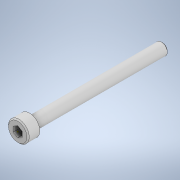
# Autodesk Inventor part: sruba
Saved by Autodesk Inventor 2020 (Build 240168000, 168)
## iProperties
Created: 2020-03-28
Part Number: sruba
Material: Ogólny
Document SubType Name: Modeling
Designer: niedz
Density: 1 g/cm^3
Appearance: Domyślna
Author: niedz
Autodesk Inventor part; units mm, degrees
ref_plane "YZ Plane" through (0, 0, 0) normal (1, 0, 0) x (0, 1, 0)
ref_plane "XZ Plane" through (0, 0, 0) normal (0, 1, 0) x (-1, 0, 0)
ref_plane "XY Plane" through (0, 0, 0) normal (0, 0, 1) x (1, 0, 0)
sketch "Szkic1" plane through (0, 0, 0) normal (0, 0, 1) x (1, 0, 0)
  circle A0 centre (0, 0) radius 3.5
  dimension "d0" = 7
  constraints: 1 centre point, 1 coincident
  measures "d0" diameter of A0
extrude "Wyciągnięcie proste1" add sketch "Szkic1" along normal blind 4
chamfer "Faza1" distance 0.4 angle 45 1 edges at (-3.5, 0, 4)
sketch "Szkic2" plane through (0, 0, 4) normal (0, 0, 1) x (1, 0, 0)
  point P0 (0, 0)
sketch "Szkic3" plane through (0, 0, 4) normal (0, 0, 1) x (1, 0, 0)
  circle A0 centre (0, 0) radius 1.5355
  line L0 (1.5355, 0) -> (1.5355, 0.8865)
  line L1 (1.5355, 0) -> (1.5355, -0.8865)
  line L2 (0.7677, -1.3298) -> (1.5355, -0.8865)
  line L3 (0.7677, -1.3298) -> (0, -1.773)
  line L4 (0.7678, 1.3298) -> (0, 1.773)
  line L5 (-0.7677, 1.3298) -> (0, 1.773)
  line L6 (-1.5355, 0) -> (-1.5355, 0.8865)
  line L7 (-0.7677, 1.3298) -> (-1.5355, 0.8865)
  line L8 (-0.7678, -1.3298) -> (0, -1.773)
  line L9 (0.7678, 1.3298) -> (1.5355, 0.8865)
  line L10 (-1.5355, 0) -> (-1.5355, -0.8865)
  line L11 (-0.7678, -1.3298) -> (-1.5355, -0.8865)
  dimension "d6" = 3.071
  constraints: 24 end point, 4 vertical, 1 coincident, 1 horizontal alignment, 1 point on line, 4 other
extrude "Wyciągnięcie proste2" cut sketch "Szkic3" against normal blind 2
sketch "Szkic4" plane through (0, 0, 0) normal (0, 0, -1) x (-1, 0, 0)
  circle A0 centre (0, 0) radius 2
  dimension "d13" = 4
  constraints: 1 centre point, 1 coincident
  measures "d13" diameter of A0
extrude "Wyciągnięcie proste3" add sketch "Szkic4" along normal blind 45
fillet "Zaokrąglenie1" radius 0.2 1 edges at (2, 0, 0)
sketch "Szkic5" plane through (0, 0, 0) normal (0, 0, -1) x (-1, 0, 0)
  point P0 (0, 0)
chamfer "Faza2" distance 0.3 angle 45 1 edges at (2, 0, -45)
sketch "Szkic6" plane through (0, 0, -45) normal (0, 0, -1) x (-1, 0, 0)
  point P0 (0, 0)
